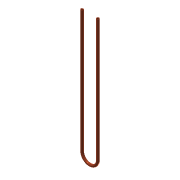
# Autodesk Inventor part: 17-0028-0022
Saved by Autodesk Inventor 2016 SP2 (Build 200236200, 236)
## iProperties
Category: IOP
Company: Universiteit van Amsterdam
Created: 2017-11-02
Part Number: 17-0028-0022
Material: Copper
Document SubType Name: Modeling
Designer: Daan Giesen
Density: 8.94 g/cm^3
Appearance: Copper - Satin
Mass: 86.5814 g
Surface Area: 194.009 cm^2
Volume: 9.68472 cm^3
Project: Digital PID Loop
Cost Center: 17-0028
User Status: Work in Progress
Authority: Reichsöllner, Lukas
Description: water cooling tube
d4: 6,000 mm
d5: 4,000 mm
d6: 36,000 mm
d7: 280,000 mm
d8: 0,00 deg
d9: 0,00 deg
Author: Daan Giesen
Title: Digital PID Loop
Revision Number: A
Autodesk Inventor part; units mm, degrees
ref_plane "YZ Plane" through (0, 0, 0) normal (1, 0, 0) x (0, 1, 0)
ref_plane "XZ Plane" through (0, 0, 0) normal (0, 1, 0) x (-1, 0, 0)
ref_plane "XY Plane" through (0, 0, 0) normal (0, 0, 1) x (1, 0, 0)
sketch "Sketch1" plane through (0, 0, 0) normal (0, 0, 1) x (1, 0, 0)
  line L0 (0, 4.2) -> (0, -4.2) construction
  line L1 (-4.2, 0) -> (4.2, 0) construction
  circle A0 centre (0, 0) radius 3
  circle A1 centre (0, 0) radius 2
  dimension "d4" = 6
  dimension "d5" = 4
  constraints: 2 centre point, 2 coincident
  measures "d4" diameter of A0
  measures "d5" diameter of A1
sketch "Sketch2" plane through (0, 0, 0) normal (0, 1, 0) x (-1, 0, 0)
  line L0 (0, 0) -> (0, -280)
  arc A0 (0, -280) -> (36, -280) centre (18, -280) ccw
  line L1 (36, -280) -> (36, 0)
  dimension "d6" = 36
  dimension "d7" = 280
  dimension "d13" = 280
  constraints: 4 end point, 2 point on circle, 2 tangent, 2 vertical, 1 centre point
  measures "d6" distance between parallel lines of L1 L0
  measures "d7" vertical distance of L1.end A0.centre
  measures "d13" distance of L0.start L0.end
sweep "Sweep1" add profiles "Sketch1" path "Sketch2"
equation "\"d7\" = d13"
body "Solid3"
